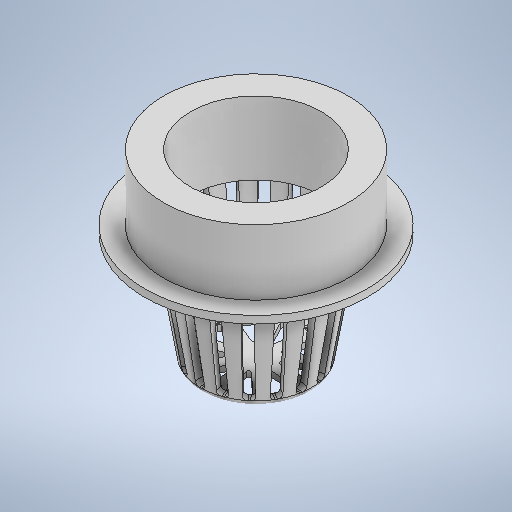
# Autodesk Inventor part: Water Sensor Grate
Saved by Autodesk Inventor 2025 (Build 290162000, 162)
## iProperties
Created: 2024-07-09
Part Number: Water Sensor Grate
Material: Generic
Document SubType Name: Modeling
Designer: track
Density: 1 g/cm^3
Appearance: Default
Author: track
Autodesk Inventor part; units mm, degrees
ref_plane "YZ Plane" through (0, 0, 0) normal (1, 0, 0) x (0, 1, 0)
ref_plane "XZ Plane" through (0, 0, 0) normal (0, 1, 0) x (-1, 0, 0)
sketch "Sketch3" plane through (0, 0, 0) normal (0, 1, 0) x (-1, 0, 0)
  circle A0 centre (0, 0) radius 35
  circle A1 centre (0, 0) radius 49.5
  dimension "d10" = 99
  dimension "d11" = 70
  constraints: 2 centre point, 2 coincident
  measures "d10" diameter of A1
  measures "d11" diameter of A0
extrude "Extrusion1" add sketch "Sketch3" against normal blind 35
sketch "Sketch4" plane through (0, -35, 0) normal (0, -1, 0) x (1, 0, 0)
  circle A0 centre (0, 0) radius 35
  circle A1 centre (0, 0) radius 59.5
  circle A2 centre (0, 0) radius 35 projected
  circle A3 centre (0, 0) radius 49.5 projected
  dimension "d14" = 10
  constraints: 2 centre point, 2 coincident, 1 concentric
  measures "d14" radial gap between concentric circles of A3 A1
extrude "Extrusion2" add sketch "Sketch4" along normal blind 4 contours A1 | A3
sketch "Sketch5" plane through (0, 0, 0) normal (0, 0, 1) x (1, 0, 0)
  line L0 (35, -39) -> (-35, -39) projected
  line L1 (0, -39) -> (0, -99) construction
  line L2 (-59.5, -39) -> (59.5, -39) projected
  line L3 (39.053, -39) -> (29.25, -99)
  line L4 (29.25, -99) -> (0, -99)
  line L5 (0, -96) -> (25.6871, -96)
  line L6 (25.6871, -96) -> (35, -39)
  line L7 (35, -39) -> (39.053, -39)
  line L8 (39.053, -39) -> (0, -39)
  line L9 (39.053, -39) -> (39.053, -99) construction
  line L10 (39.053, -99) -> (29.25, -99) construction
  line L11 (0, -99) -> (0, -96)
  line L12 (0, -39) -> (35, -39)
  point P0 (0, 0)
  point P1 (34, -39)
  dimension "d17" = 3
  dimension "d18" = 4
  dimension "d21" = 60
  dimension "d23" = 29.25
  constraints: 22 end point, 3 collinear, 2 horizontal, 2 perpendicular, 2 point on line, 2 vertical, 1 midpoint, 1 parallel
  measures "d17" distance between parallel lines of L4 L5
  measures "d18" distance between parallel lines of L3 L6
  measures "d21" distance of L1.start L1.end
  measures "d23" distance of L3.end L1.end
revolve "Revolution2" add sketch "Sketch5" angle 360 about axis through (0, -39, 0) along (0, -1, 0)
ref_plane "Work Plane1" through (0, 0, 49.5) normal (0, 0, 1) x (1, 0, 0)
fillet "Fillet1" radius 4 1 edges at (-29.25, -99, 0)
sketch "Sketch7" plane through (0, -99, 0) normal (0, -1, 0) x (1, 0, 0)
  line L0 (0, 0) -> (-25.8505, 0) construction
  circle A0 centre (0, 0) radius 25.8505 projected
  line L1 (-10.4952, -0.953) -> (-23.4952, -5.0858)
  line L2 (-24.7982, -4.1328) -> (-24.7982, 4.1328)
  line L3 (-23.4952, 5.0858) -> (-10.4952, 0.953)
  circle A1 centre (0, 0) radius 29.7982 projected
  arc A2 (-23.4952, 5.0858) -> (-24.7982, 4.1328) centre (-23.7982, 4.1328) ccw
  arc A3 (-24.7982, -4.1328) -> (-23.4952, -5.0858) centre (-23.7982, -4.1328) ccw
  arc A4 (-10.4952, -0.953) -> (-10.4952, 0.953) centre (-10.7982, 0) ccw
  point P0 (-7.4974, 0)
  point P1 (-24.7982, -5.5)
  point P2 (-24.7982, 5.5)
  point P3 (-9.7982, 0)
  dimension "d26" = 11
  dimension "d28" = 5
  dimension "d29" = 1
  dimension "d30" = 15
  constraints: 8 end point, 7 point on circle, 7 point on line, 6 tangent, 3 centre point, 2 equal radius, 1 horizontal, 1 horizontal alignment, 1 vertical, 2 other
  measures "d26" distance of point (-24.798, -5.5) point (-24.798, 5.5)
  measures "d28" distance edge to line of A1 L2
  measures "d29" radius of A2
  measures "d30" distance from line of point (-9.798, 0) L2
extrude "Extrusion3" cut sketch "Sketch7" against normal blind 4 contours L1 A3 L2 A2 L3 A4
pattern_circular "Circular Pattern1" count 9 over 360 about axis through (0, -95, 0) along (0, -1, 0) of "Extrusion3"
sketch "Sketch8" plane through (0, 0, 49.5) normal (0, 0, 1) x (1, 0, 0)
  line L0 (-29.7982, -95.645) -> (29.7982, -95.645) projected
  line L1 (0, -95.645) -> (0, -39) construction
  line L2 (35, -39) -> (-35, -39) projected
  line L3 (2.5, -39) -> (-2.5, -39)
  line L4 (-2.5, -39) -> (-2.5, -93.645)
  line L5 (-0.5, -95.645) -> (0.5, -95.645)
  line L6 (2.5, -93.645) -> (2.5, -39)
  line L7 (2.5, -39) -> (-2.5, -95.645) construction
  line L8 (-2.5, -39) -> (2.5, -95.645) construction
  arc A0 (-2.5, -93.645) -> (-0.5, -95.645) centre (-0.5, -93.645) ccw
  arc A1 (0.5, -95.645) -> (2.5, -93.645) centre (0.5, -93.645) ccw
  point P0 (0, 0)
  point P1 (0, -67.3225)
  point P2 (-2.5, -39)
  dimension "d36" = 5
  dimension "d37" = 2
  constraints: 14 end point, 5 midpoint, 5 point on line, 4 point on circle, 4 tangent, 2 centre point, 2 parallel, 1 equal radius, 1 horizontal, 1 perpendicular
  measures "d36" distance between parallel lines of L6 L4
  measures "d37" radius of A0
extrude "Extrusion4" cut sketch "Sketch8" against normal up to surface
pattern_circular "Circular Pattern2" count 18 over 360 about axis through (0, -69, 0) along (0, -1, 0) of "Extrusion4"
body "Solid2"
